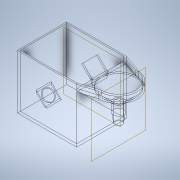
# Autodesk Inventor part: Resoar V2
Saved by Autodesk Inventor 2021 (Build 250183000, 183)
## iProperties
Created: 2025-01-08
Part Number: Resoar V2
Material: Generic
Document SubType Name: Modeling
Designer: 24lucsil
Density: 1 g/cm^3
Appearance: Default
Author: 24lucsil
Autodesk Inventor part; units mm, degrees
ref_plane "YZ Plane" through (0, 0, 0) normal (1, 0, 0) x (0, 1, 0)
ref_plane "XZ Plane" through (0, 0, 0) normal (0, 1, 0) x (-1, 0, 0)
ref_plane "XY Plane" through (0, 0, 0) normal (0, 0, 1) x (1, 0, 0)
sketch "Sketch1" plane through (0, 0, 0) normal (0, 1, 0) x (-1, 0, 0)
  line L0 (0, 0) -> (-120, 0)
  line L1 (-120, 0) -> (-120, -100)
  line L2 (-120, -100) -> (0, -100)
  line L3 (0, -100) -> (0, 0)
  dimension "d0" = 120
  dimension "d1" = 100
  constraints: 8 end point, 2 parallel, 1 horizontal, 1 perpendicular
  measures "d0" distance of L0.start L0.end
  measures "d1" distance of L2.end L0.start
extrude "Extrusion1" add sketch "Sketch1" along normal blind 3
sketch "Sketch2" plane through (0, 3, 0) normal (0, 1, 0) x (1, 0, 0)
  line L0 (0, 100) -> (0, 0) construction
  line L1 (0, 0) -> (3, 0) construction
  line L2 (3, 0) -> (3, 3) construction
  line L3 (3, 3) -> (0, 3) construction
  line L4 (0, 3) -> (0, 0) construction
  line L5 (120, 100) -> (0, 100) construction
  line L6 (120, 100) -> (117, 100) construction
  line L7 (117, 100) -> (117, 97) construction
  line L8 (117, 97) -> (120, 97) construction
  line L9 (120, 97) -> (120, 100) construction
  line L10 (3, 3) -> (117, 3)
  line L11 (117, 3) -> (117, 97)
  line L12 (117, 97) -> (3, 97)
  line L13 (3, 97) -> (3, 3)
  line L14 (120, 0) -> (120, 100) projected
  line L15 (0, 0) -> (120, 0)
  line L16 (120, 0) -> (120, 100)
  line L17 (120, 100) -> (0, 100)
  line L18 (0, 100) -> (0, 0)
  dimension "d4" = 3
  dimension "d5" = 3
  dimension "d6" = 3
  dimension "d7" = 3
  constraints: 32 end point, 8 parallel, 4 horizontal, 4 perpendicular
  measures "d4" distance of L6.end L7.end
  measures "d5" distance of L7.end L8.end
  measures "d6" distance of L2.end L3.end
  measures "d7" distance of L1.end L2.end
extrude "Extrusion2" add sketch "Sketch2" along normal blind 97
ref_plane "Work Plane1" through (155, 0, 0) normal (1, 0, 0) x (0, 0, -1)
sketch "Sketch3" plane through (155, 0, 0) normal (1, 0, 0) x (0, 0, -1)
  line L0 (0, 0) -> (0, 100) construction
  line L1 (0, 0) -> (50, 0) construction
  line L2 (100, 0) -> (0, 0) construction
  line L3 (50, 0) -> (50, 35) construction
  line L4 (50, 35) -> (43, 35) construction
  line L5 (50, 35) -> (50, 73) construction
  line L6 (50, 73) -> (40, 73) construction
  line L7 (40, 73) -> (40, 54) construction
  line L8 (43, 35) -> (40, 54)
  line L9 (43, 35) -> (43, 73)
  line L10 (40, 54) -> (40, 73)
  line L11 (3, 100) -> (97, 100) construction
  line L12 (50, 100) -> (15, 100) construction
  line L13 (15, 100) -> (15, 97)
  line L14 (15, 97) -> (40, 73)
  line L15 (15, 100) -> (43, 73)
  dimension "d11" = 35
  dimension "d12" = 7
  dimension "d13" = 38
  dimension "d14" = 10
  dimension "d15" = 35
  dimension "d16" = 3
  constraints: 26 end point, 4 vertical, 3 point on line, 2 midpoint, 2 perpendicular, 1 collinear, 1 horizontal
  measures "d11" distance of L1.end L3.end
  measures "d12" distance of L3.end L4.end
  measures "d13" distance of L3.end L5.end
  measures "d14" distance of L5.end L6.end
  measures "d15" distance of L12.end L12.start
  measures "d16" distance of L12.end L13.end
revolve "Revolution1" add sketch "Sketch3" angle 360 about axis through (155, 35, -50) along (0, 1, 0)
sketch "Sketch4" plane through (0, 100, 0) normal (0, 1, 0) x (1, 0, 0)
  line L0 (120, 0) -> (120, 100) projected
  line L1 (120, 0) -> (120, 3)
  line L2 (120, 100) -> (0, 100) projected
  line L3 (120, 100) -> (120, 97)
  line L4 (120, 97) -> (155, 85)
  circle A0 centre (155, 50) radius 35 projected
  line L5 (155, 15) -> (120, 3)
  line L6 (120, 97) -> (120, 3)
  arc A1 (155, 85) -> (155, 15) centre (155, 50) ccw
  line L7 (120, 100) -> (159.5039, 86.4558)
  line L8 (120, 0) -> (154.2885, 10.5356)
  line L9 (155, 50) -> (194, 50) construction
  arc A2 (154.2885, 10.5356) -> (159.5039, 86.4558) centre (155.9663, 48.5596) ccw
  arc A3 (155, 15) -> (155, 85) centre (155, 50) ccw
  point P0 (0, 0)
  dimension "d18" = 3
  dimension "d19" = 3
  dimension "d20" = 39
  constraints: 16 end point, 9 point on circle, 3 centre point, 2 concentric, 2 point on line, 1 horizontal, 1 parallel, 1 vertical
  measures "d18" distance of L1.end L0.start
  measures "d19" distance of L0.end L3.end
  measures "d20" distance of L9.start L9.end
extrude "Extrusion3" add sketch "Sketch4" against normal blind 3 contours L0 L5 A0 L4 L7 A2 L8 | L0 A0 L5 | L0 L4 A0
sketch "Sketch5" plane through (0, 100, 0) normal (0, 1, 0) x (1, 0, 0)
  line L0 (120, 0) -> (120, 100) projected
  line L1 (0, 100) -> (0, 0) projected
  line L2 (120, 0) -> (0, 0)
  line L3 (0, 0) -> (0, 100)
  line L4 (0, 100) -> (120, 100)
  line L5 (120, 100) -> (120, 0)
  arc A0 (154.2885, 10.5356) -> (159.5039, 86.4558) centre (155.9663, 48.5596) ccw projected
  line L6 (120, 100) -> (159.5039, 86.4558) projected
  arc A1 (154.2885, 10.5356) -> (159.5039, 86.4558) centre (157.8261, 48.4318) ccw
  circle A2 centre (155, 50) radius 35 projected
  arc A3 (155, 15) -> (155, 85) centre (155, 50) ccw
  line L7 (117, 3) -> (117, 97) projected
  line L8 (155, 85) -> (117, 97)
  line L9 (155, 15) -> (117, 3)
  line L10 (120, 100) -> (156.887, 86.4812)
  line L11 (154.2885, 10.5356) -> (120, 0) projected
  line L12 (154.2885, 10.5356) -> (120, 0)
  line L13 (117, 3) -> (3, 3) projected
  line L14 (3, 3) -> (3, 97) projected
  line L15 (117, 3) -> (3, 3)
  line L16 (3, 3) -> (3, 97)
  line L17 (3, 97) -> (117, 97)
  line L18 (117, 97) -> (117, 3)
  point P0 (117, 97)
  constraints: 24 end point, 7 point on circle, 4 parallel, 2 centre point, 2 horizontal, 2 perpendicular
extrude "Extrusion4" add sketch "Sketch5" along normal blind 10 contours L2 L1 L4 L0 L8 L17 L14 L13 L9 | L0 L9 A2 L8 L6 A0 L11
ref_plane "Work Plane2" through (3, 3, -65) normal (0, 0, 1) x (1, 0, 0)
sketch "Sketch6" plane through (3, 3, -65) normal (0, 0, 1) x (1, 0, 0)
  line L0 (0, 0) -> (0, 107) projected
  line L1 (0, 0) -> (0, 21.21)
  line L2 (0, 0) -> (114, 0) projected
  line L3 (0, 0) -> (21.21, 0)
  line L4 (114, 0) -> (0, 0) projected
  line L5 (0, 21.21) -> (21.21, 0)
  line L6 (0, 21.21) -> (0, 17.21)
  line L7 (0, 17.21) -> (17.21, 0)
  point P0 (-3, -3)
  point P1 (0, 17.21)
  point P2 (17.21, 0)
  point P3 (21.21, 0)
  dimension "d26" = 21.21
  dimension "d27" = 21.21
  dimension "d28" = 4
  constraints: 10 end point, 4 point on line, 1 parallel
  measures "d26" distance from line of L2 L1.end
  measures "d27" distance of L0.start L3.end
  measures "d28" distance of L6.end L1.end
extrude "Extrusion5" add sketch "Sketch6" along normal blind 30 contours L0 L5 L2 L7
sketch "Sketch7" plane through (3, 24.21, -65) normal (0.7071068, 0.7071068, 0) x (-0.7071068, 0.7071068, 0)
  line L0 (-29.9955, 30) -> (0, 30) projected
  line L1 (-14.9977, 30) -> (-14.9977, 15)
  circle A0 centre (-14.9977, 15) radius 11
  point P0 (-14.9977, 65)
  dimension "d31" = 15
  dimension "d32" = 22
  constraints: 2 end point, 1 centre point, 1 coincident, 1 midpoint, 1 vertical
  measures "d31" distance of L1.start L1.end
  measures "d32" diameter of A0
extrude "Extrusion6" cut sketch "Sketch7" against normal blind 3.6
sketch "Sketch11" plane through (3, 3, -65) normal (0, 0, 1) x (1, 0, 0)
  line L0 (18.3832, 2.8268) -> (16.3832, 0.8268) construction
  line L1 (18.3832, 2.8268) -> (148.3832, 132.8268) construction
  line L2 (2.8268, 18.3832) -> (0.8268, 16.3832) construction
  line L3 (2.8268, 18.3832) -> (132.8268, 148.3832) construction
  line L4 (113.4034, 97.847) -> (95.0186, 116.2318) construction
  line L5 (95.0186, 116.2318) -> (92.0186, 113.2318) construction
  line L6 (92.0186, 113.2318) -> (113.4034, 91.847) construction
  line L7 (117, 97) -> (145, 70) projected
  line L8 (117, 97) -> (113.4034, 97.847)
  line L9 (113.4034, 97.847) -> (95.0186, 116.2318)
  line L10 (95.0186, 116.2318) -> (92.0186, 113.2318)
  line L11 (92.0186, 113.2318) -> (110.4034, 94.847)
  line L12 (110.4034, 94.847) -> (114, 85.1798)
  line L13 (114, 0) -> (114, 97) projected
  line L14 (114, 85.1798) -> (117, 85.1798)
  line L15 (117, 85.1798) -> (117, 97)
  line L16 (117, 94) -> (117, 107) projected
  point P0 (-3, -3)
  dimension "d65" = 130
  dimension "d66" = 130
  dimension "d67" = 26
  dimension "d68" = 3
  dimension "d69" = 134.3788
  dimension "d70" = 4.2426
  dimension "d71" = 49.4689
  dimension "d72" = 49.4689
  dimension "d73" = 25.634
  dimension "d74" = 149.293
  dimension "d75" = 0
  constraints: 24 end point, 7 point on line, 4 collinear, 3 perpendicular, 2 parallel
  measures "d65" horizontal distance of L3.start L3.end
  measures "d66" horizontal distance of L1.start L1.end
  measures "d67" distance of L4.start L4.end
  measures "d68" horizontal distance of L4.end L5.end
  measures "d69" distance from line of L0.start L4
  measures "d70" distance from line of L6.end L0
  measures "d71" distance from line of L1.end L4
  measures "d72" distance from line of L3.end L4
  measures "d73" angle of L7 L12
  measures "d74" angle of L8 L7
  measures "d75" distance between parallel lines of L15 L16
extrude "Extrusion8" add sketch "Sketch11" along normal blind 30
body "Solid1"
